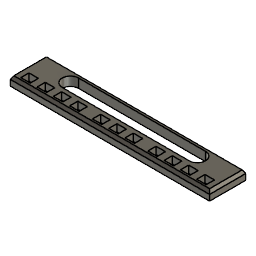
Smart Fan Shroud (Autodesk Fusion 360 design; units mm, degrees)
part number: 2026-06-19-12-40-10-086
Autodesk Fusion 360 part; units mm, degrees
sketch "Sketch1" plane through (0, 0, 0) normal (0, 0, 1) x (1, 0, 0)
  line L0 (0, 0) -> (110, 0)
  line L1 (110, 0) -> (110, 20)
  line L2 (110, 20) -> (0, 20)
  line L3 (0, 20) -> (0, 0)
  dimension "d1" = 110
  dimension "d2" = 20
  constraint horizontal L0
  constraint vertical L1
  constraint horizontal L2
  constraint vertical L3
  constraint coincident L0.start L3.end
  measures "d1" distance of L0.start L0.end
  measures "d2" distance of L0.start L2.end
extrude "Extrude1" add sketch "Sketch1" along normal blind 5
sketch "Sketch2" plane through (0, 0, 5) normal (0, 0, 1) x (-1, 0, 0)
  line L0 (0, -20) -> (0, 0)
  line L1 (0, 0) -> (-110, 0)
  line L2 (-110, 0) -> (-110, -20)
  line L3 (-110, -20) -> (0, -20)
  line L4 (-3.85, -2) -> (-106.15, -2) construction
  line L5 (-46, -2) -> (-46, -6.5) construction
  line L6 (-91.95, -6.5) -> (-91.95, -2)
  line L7 (-97.15, -6.5) -> (-91.95, -6.5)
  line L8 (-73.95, -6.5) -> (-73.95, -2)
  line L9 (-55, -2) -> (-55, -6.5) construction
  line L10 (-33.45, -2) -> (-33.45, -6.5) construction
  line L11 (-27.05, -2) -> (-27.05, -6.5)
  line L12 (-30.85, -6.5) -> (-30.85, -2)
  line L13 (-43.4, -6.5) -> (-43.4, -2)
  line L14 (-18.05, -2) -> (-18.05, -6.5)
  line L15 (-21.85, -6.5) -> (-21.85, -2)
  line L16 (-36.05, -6.5) -> (-30.85, -6.5)
  line L17 (-9.05, -2) -> (-9.05, -6.5)
  line L18 (-9.05, -6.5) -> (-3.85, -6.5)
  line L19 (-21.85, -2) -> (-27.05, -2)
  line L20 (-3.85, -2) -> (-9.05, -2)
  line L21 (-12.85, -2) -> (-18.05, -2)
  line L22 (-3.85, -6.5) -> (-3.85, -2)
  line L23 (-18.05, -6.5) -> (-12.85, -6.5)
  line L24 (-30.85, -2) -> (-36.05, -2)
  line L25 (-82.95, -6.5) -> (-82.95, -2)
  line L26 (-57.6, -2) -> (-57.6, -6.5)
  line L27 (-48.6, -2) -> (-48.6, -6.5)
  line L28 (-61.4, -2) -> (-66.6, -2)
  line L29 (-64, -2) -> (-64, -6.5) construction
  line L30 (-106.15, -6.5) -> (-100.95, -6.5)
  line L31 (-100.95, -2) -> (-106.15, -2)
  line L32 (-106.15, -2) -> (-106.15, -6.5)
  line L33 (-79.15, -2) -> (-79.15, -6.5)
  line L34 (-61.4, -6.5) -> (-61.4, -2)
  line L35 (-52.4, -6.5) -> (-52.4, -2)
  line L36 (-88.15, -6.5) -> (-82.95, -6.5)
  line L37 (-97.15, -2) -> (-97.15, -6.5)
  line L38 (-106.15, -2) -> (-106.15, -6.5) construction
  line L39 (-48.6, -6.5) -> (-43.4, -6.5)
  line L40 (-52.4, -2) -> (-57.6, -2)
  line L41 (-76.55, -2) -> (-76.55, -6.5) construction
  line L42 (-43.4, -2) -> (-48.6, -2)
  line L43 (-57.6, -6.5) -> (-52.4, -6.5)
  line L44 (-66.6, -6.5) -> (-61.4, -6.5)
  line L45 (-82.95, -2) -> (-88.15, -2)
  line L46 (-66.6, -2) -> (-66.6, -6.5)
  line L47 (-100.95, -6.5) -> (-100.95, -2)
  line L48 (-91.95, -2) -> (-97.15, -2)
  line L49 (-88.15, -2) -> (-88.15, -6.5)
  line L50 (-27.05, -6.5) -> (-21.85, -6.5)
  line L51 (-12.85, -6.5) -> (-12.85, -2)
  line L52 (-36.05, -2) -> (-36.05, -6.5)
  line L53 (-3.85, -6.5) -> (-3.85, -2) construction
  line L54 (-73.95, -2) -> (-79.15, -2)
  line L55 (-106.15, -6.5) -> (-3.85, -6.5) construction
  line L56 (-79.15, -6.5) -> (-73.95, -6.5)
  line L57 (0, -2) -> (-110, -2) construction
  line L58 (-55, -20) -> (-55, 0) construction
  dimension "d27" = 9
  dimension "d28" = 0
  dimension "d31" = 9
  dimension "d32" = 0
  dimension "d35" = 9
  dimension "d36" = 0
  dimension "d37" = 5.2
  dimension "d38" = 4.5
  dimension "d39" = 5.2
  dimension "d40" = 4.5
  dimension "d41" = 12.55
  dimension "d42" = 5.2
  dimension "d43" = 4.5
  dimension "d44" = 12.55
  dimension "d45" = 2
  constraint horizontal L30
  constraint vertical L47
  constraint horizontal L31
  constraint vertical L32
  constraint midpoint L41.start L54
  constraint midpoint L41.end L56
  constraint horizontal L44
  constraint vertical L34
  constraint horizontal L28
  constraint vertical L46
  constraint midpoint L29.start L28
  constraint midpoint L29.end L44
  constraint collinear L28 L54
  constraint horizontal L16
  constraint vertical L12
  constraint horizontal L24
  constraint vertical L52
  constraint midpoint L10.start L24
  constraint midpoint L10.end L16
  constraint midpoint L5.start L42
  constraint midpoint L5.end L39
  constraint collinear L24 L42
  constraint horizontal L55
  constraint vertical L53
  constraint horizontal L4
  constraint vertical L38
  constraint midpoint L9.start L4
  constraint midpoint L9.end L55
  constraint collinear L4 L31
  constraint collinear L32 L38
  constraint collinear L30 L55
  constraint collinear L22 L53
  constraint coincident L0 L57.start
  constraint coincident L2 L57.end
  constraint perpendicular L2 L57
  constraint midpoint L3 L58.start
  constraint midpoint L1 L58.end
  constraint collinear L9 L58
  constraint collinear L40 L57
  measures "d37" distance of L30.end L30.start
  measures "d38" distance of L4.end L30.start
  measures "d39" distance of L34.start L44.start
  measures "d40" distance of L28.end L44.start
  measures "d41" distance of L29 L41
  measures "d42" distance of L12.start L16.start
  measures "d43" distance of L24.end L16.start
  measures "d44" distance of L5 L10
  measures "d45" distance of L1 L57
extrude "Extrude2" cut sketch "Sketch2" against normal blind 4 contours L6 L7 L37 L48 | L8 L33 L54 L56 | L11 L15 L19 L50 | L12 L16 L24 L52 | L13 L27 L39 L42 | L14 L21 L23 L51 | L17 L18 L20 L22 | L25 L36 L45 L49 | L26 L35 L40 L43 | L28 L34 L44 L46 | L30 L31 L32 L47
sketch "Sketch3" plane through (0, 0, 1) normal (0, 0, 1) x (-1, 0, 0)
  line L0 (-3.85, -6.5) -> (-3.85, -2)
  line L1 (-3.85, -2) -> (-9.05, -2)
  line L2 (-9.05, -2) -> (-9.05, -6.5)
  line L3 (-9.05, -6.5) -> (-3.85, -6.5)
  line L4 (-4.35, -6) -> (-8.55, -6)
  line L5 (-8.55, -6) -> (-8.55, -2.5)
  line L6 (-8.55, -2.5) -> (-4.35, -2.5)
  line L7 (-4.35, -2.5) -> (-4.35, -6)
  line L8 (-13.35, -6) -> (-17.55, -6)
  line L9 (-17.55, -6) -> (-17.55, -2.5)
  line L10 (-17.55, -2.5) -> (-13.35, -2.5)
  line L11 (-13.35, -2.5) -> (-13.35, -6)
  line L12 (-22.35, -6) -> (-26.55, -6)
  line L13 (-26.55, -6) -> (-26.55, -2.5)
  line L14 (-26.55, -2.5) -> (-22.35, -2.5)
  line L15 (-22.35, -2.5) -> (-22.35, -6)
  line L16 (-31.35, -6) -> (-35.55, -6)
  line L17 (-35.55, -6) -> (-35.55, -2.5)
  line L18 (-35.55, -2.5) -> (-31.35, -2.5)
  line L19 (-31.35, -2.5) -> (-31.35, -6)
  line L20 (-43.9, -6) -> (-48.1, -6)
  line L21 (-48.1, -6) -> (-48.1, -2.5)
  line L22 (-48.1, -2.5) -> (-43.9, -2.5)
  line L23 (-43.9, -2.5) -> (-43.9, -6)
  line L24 (-43.4, -6.5) -> (-48.6, -6.5)
  line L25 (-48.6, -2) -> (-43.4, -2)
  line L26 (-48.6, -6.5) -> (-48.6, -2)
  line L27 (-43.4, -2) -> (-43.4, -6.5)
  line L28 (-52.9, -6) -> (-57.1, -6)
  line L29 (-57.1, -6) -> (-57.1, -2.5)
  line L30 (-57.1, -2.5) -> (-52.9, -2.5)
  line L31 (-52.9, -2.5) -> (-52.9, -6)
  line L32 (-61.9, -6) -> (-66.1, -6)
  line L33 (-66.1, -6) -> (-66.1, -2.5)
  line L34 (-66.1, -2.5) -> (-61.9, -2.5)
  line L35 (-61.9, -2.5) -> (-61.9, -6)
  line L36 (-78.65, -2.5) -> (-74.45, -2.5)
  line L37 (-78.65, -6) -> (-78.65, -2.5)
  line L38 (-74.45, -6) -> (-78.65, -6)
  line L39 (-74.45, -2.5) -> (-74.45, -6)
  line L40 (-73.95, -6.5) -> (-79.15, -6.5)
  line L41 (-79.15, -2) -> (-73.95, -2)
  line L42 (-79.15, -6.5) -> (-79.15, -2)
  line L43 (-73.95, -2) -> (-73.95, -6.5)
  line L44 (-87.65, -6) -> (-87.65, -2.5)
  line L45 (-87.65, -2.5) -> (-83.45, -2.5)
  line L46 (-83.45, -2.5) -> (-83.45, -6)
  line L47 (-83.45, -6) -> (-87.65, -6)
  line L48 (-96.65, -6) -> (-96.65, -2.5)
  line L49 (-96.65, -2.5) -> (-92.45, -2.5)
  line L50 (-92.45, -2.5) -> (-92.45, -6)
  line L51 (-92.45, -6) -> (-96.65, -6)
  line L52 (-105.65, -6) -> (-105.65, -2.5)
  line L53 (-105.65, -2.5) -> (-101.45, -2.5)
  line L54 (-101.45, -2.5) -> (-101.45, -6)
  line L55 (-101.45, -6) -> (-105.65, -6)
  dimension "d48" = 0.5
  dimension "d49" = 0.5
  dimension "d50" = 0.5
  dimension "d51" = 0.5
  dimension "d54" = -9
  dimension "d55" = 0
  dimension "d56" = 0.5
  dimension "d57" = 0.5
  dimension "d58" = 0.5
  dimension "d59" = 0.5
  dimension "d62" = -9
  dimension "d63" = 0
  dimension "d64" = 0.5
  dimension "d65" = 0.5
  dimension "d66" = 0.5
  dimension "d67" = 0.5
  dimension "d70" = -9
  dimension "d71" = 0
  constraint horizontal L4
  constraint vertical L5
  constraint horizontal L6
  constraint vertical L7
  constraint horizontal L20
  constraint vertical L21
  constraint horizontal L22
  constraint vertical L23
  constraint horizontal L38
  constraint vertical L37
  constraint horizontal L36
  constraint vertical L39
  measures "d48" distance of L3 L4
  measures "d49" distance of L2 L5
  measures "d50" distance of L1 L6
  measures "d51" distance of L0 L7
  measures "d56" distance of L20 L24
  measures "d57" distance of L22 L25
  measures "d58" distance of L21 L26
  measures "d59" distance of L23 L27
  measures "d64" distance of L38 L40
  measures "d65" distance of L36 L41
  measures "d66" distance of L37 L42
  measures "d67" distance of L39 L43
extrude "Extrude3" cut sketch "Sketch3" against normal blind 2 contours L4 L5 L6 L7 | L8 L9 L10 L11 | L12 L13 L14 L15 | L16 L17 L18 L19 | L20 L21 L22 L23 | L28 L29 L30 L31 | L32 L33 L34 L35 | L36 L37 L38 L39 | L44 L45 L46 L47 | L48 L49 L50 L51 | L52 L53 L54 L55
sketch "Sketch4" plane through (0, 0, 5) normal (0, 0, 1) x (-1, 0, 0)
  line L0 (0, -20) -> (0, 0)
  line L1 (0, 0) -> (-110, 0)
  line L2 (-110, 0) -> (-110, -20)
  line L3 (-110, -20) -> (0, -20)
  line L4 (-106.15, -2) -> (-100.95, -2)
  line L5 (-100.95, -2) -> (-100.95, -6.5)
  line L6 (-100.95, -6.5) -> (-106.15, -6.5)
  line L7 (-106.15, -6.5) -> (-106.15, -2)
  line L8 (-61.4, -6.5) -> (-66.6, -6.5)
  line L9 (-66.6, -6.5) -> (-66.6, -2)
  line L10 (-66.6, -2) -> (-61.4, -2)
  line L11 (-61.4, -2) -> (-61.4, -6.5)
  line L12 (-21.85, -2) -> (-21.85, -6.5)
  line L13 (-21.85, -6.5) -> (-27.05, -6.5)
  line L14 (-27.05, -6.5) -> (-27.05, -2)
  line L15 (-27.05, -2) -> (-21.85, -2)
  line L16 (-18.05, -2) -> (-12.85, -2)
  line L17 (-12.85, -2) -> (-12.85, -6.5)
  line L18 (-12.85, -6.5) -> (-18.05, -6.5)
  line L19 (-18.05, -6.5) -> (-18.05, -2)
  line L20 (-52.4, -2) -> (-52.4, -6.5)
  line L21 (-52.4, -6.5) -> (-57.6, -6.5)
  line L22 (-57.6, -6.5) -> (-57.6, -2)
  line L23 (-57.6, -2) -> (-52.4, -2)
  line L24 (-97.15, -6.5) -> (-97.15, -2)
  line L25 (-97.15, -2) -> (-91.95, -2)
  line L26 (-91.95, -2) -> (-91.95, -6.5)
  line L27 (-91.95, -6.5) -> (-97.15, -6.5)
  line L28 (-73.95, -2) -> (-73.95, -6.5)
  line L29 (-73.95, -6.5) -> (-79.15, -6.5)
  line L30 (-79.15, -6.5) -> (-79.15, -2)
  line L31 (-79.15, -2) -> (-73.95, -2)
  line L32 (-30.85, -6.5) -> (-36.05, -6.5)
  line L33 (-36.05, -6.5) -> (-36.05, -2)
  line L34 (-36.05, -2) -> (-30.85, -2)
  line L35 (-30.85, -2) -> (-30.85, -6.5)
  line L36 (-9.05, -2) -> (-3.85, -2)
  line L37 (-3.85, -2) -> (-3.85, -6.5)
  line L38 (-3.85, -6.5) -> (-9.05, -6.5)
  line L39 (-9.05, -6.5) -> (-9.05, -2)
  line L40 (-48.6, -6.5) -> (-48.6, -2)
  line L41 (-48.6, -2) -> (-43.4, -2)
  line L42 (-43.4, -2) -> (-43.4, -6.5)
  line L43 (-43.4, -6.5) -> (-48.6, -6.5)
  line L44 (-82.95, -6.5) -> (-88.15, -6.5)
  line L45 (-88.15, -6.5) -> (-88.15, -2)
  line L46 (-88.15, -2) -> (-82.95, -2)
  line L47 (-82.95, -2) -> (-82.95, -6.5)
  line L48 (-21.85, -6.5) -> (-18.05, -6.5) construction
  line L49 (-19.95, -6.5) -> (-19.95, -20) construction
  line L50 (-88.15, -6.5) -> (-91.95, -6.5) construction
  line L51 (-90.05, -6.5) -> (-90.05, -20) construction
  circle A0 centre (-19.95, -13.25) radius 4.5
  circle A1 centre (-90.05, -13.25) radius 4.5
  line L52 (-19.95, -17.75) -> (-90.05, -17.75)
  line L53 (-90.05, -8.75) -> (-19.95, -8.75)
  dimension "d80" = 9
  dimension "d81" = 9
  constraint coincident L12.end L13.start
  constraint coincident L18.end L19.start
  constraint midpoint L48 L49.start
  constraint coincident L3 L49.end
  constraint perpendicular L3 L49
  constraint coincident L44.end L45.start
  constraint coincident L26.end L27.start
  constraint midpoint L50 L51.start
  constraint coincident L3 L51.end
  constraint perpendicular L3 L51
  constraint midpoint L49 A0.centre
  constraint midpoint L51 A1.centre
  constraint coincident A0 L52.start
  constraint coincident L49 L52.start
  constraint coincident L51 L52.end
  constraint coincident A1 L52.end
  constraint coincident A1 L53.start
  constraint coincident L51 L53.start
  constraint coincident L49 L53.end
  constraint coincident A0 L53.end
  measures "d80" diameter of A0
  measures "d81" diameter of A1
extrude "Extrude4" cut sketch "Sketch4" against normal blind 5 contours A0 | A0 A1 L52 L53 | A1
chamfer "Chamfer1" distance 1 angle 60 4 edges at (55, 20, 5) (0, 10, 5) (55, 0, 5) (110, 10, 5) measured on face at (101.8291, 13.3621, 5) measured on face at (101.8291, 13.3621, 5) measured on face at (101.8291, 13.3621, 5) measured on face at (101.8291, 13.3621, 5)
equation "d37 = 5 mm + 0.2 mm"
equation "d38 = 4.3 mm + 0.2 mm"
